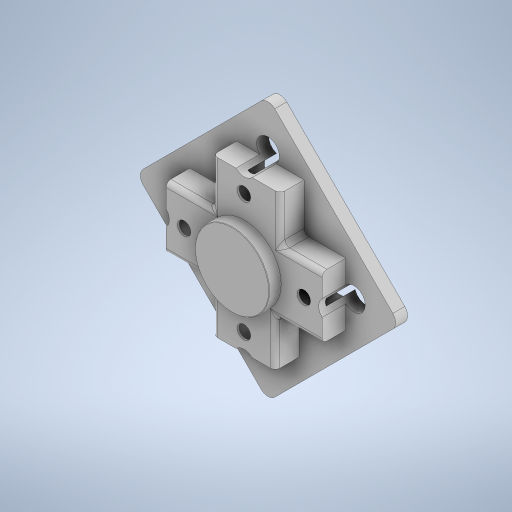
# Autodesk Inventor part: adapter_final2
Saved by Autodesk Inventor 2024 (Build 280153000, 153)
## iProperties
Created: 2024-05-24
Part Number: adapter_final2
Material: Generic
Document SubType Name: Modeling
Designer: maint
Density: 1 g/cm^3
Appearance: Default
Author: maint
Autodesk Inventor part; units mm, degrees
ref_plane "YZ Plane" through (0, 0, 0) normal (1, 0, 0) x (0, 1, 0)
ref_plane "XZ Plane" through (0, 0, 0) normal (0, 1, 0) x (-1, 0, 0)
ref_plane "XY Plane" through (0, 0, 0) normal (0, 0, 1) x (1, 0, 0)
sketch "Sketch1" plane through (0, 0, 0) normal (0, 0, 1) x (1, 0, 0)
  line L0 (41, -41) -> (-41, -41)
  line L1 (-41, -41) -> (-41, 41)
  line L2 (-41, 41) -> (41, 41)
  line L3 (41, 41) -> (41, -41)
  line L4 (41, -41) -> (-41, 41) construction
  line L5 (-41, -41) -> (41, 41) construction
  line L6 (-55, 0) -> (0, 55)
  line L7 (0, 55) -> (55, 0)
  line L8 (55, 0) -> (0, -55)
  line L9 (0, -55) -> (-55, 0)
  line L10 (-55, 0) -> (55, 0)
  line L11 (0, 55) -> (0, -55)
  circle A0 centre (0, 0) radius 63.5
  point P0 (-41, 0)
  dimension "d0" = 82
  dimension "d86" = 110
  dimension "d87" = 0
  dimension "d88" = 110
  dimension "d89" = 0
  dimension "d93" = 127
  constraints: 24 end point, 4 midpoint, 4 parallel, 3 perpendicular, 1 centre point, 1 coincident, 1 horizontal
  measures "d0" distance of L1.end L2.end
  measures "d86" distance of L8.end L6.end
  measures "d87" vertical distance of L7.end L6.start
  measures "d88" distance of L7.end L6.start
  measures "d89" distance from line of point (-41, 0) L10
  measures "d93" diameter of A0
extrude "Extrusion1" add sketch "Sketch1" along normal blind 15 contours L8 L11 L0 | L0 L11 L10 L3 L8 | L3 L10 L8 | L11 L9 L0 | L0 L9 L1 L10 L11 | L10 L11 L2 L7 L3 | L3 L7 L10 | L10 L1 L6 L2 L11 | L9 L10 L1 | L10 L6 L1 | L11 L7 L2 | L2 L6 L11
sketch "Sketch2" plane through (0, 0, 0) normal (0, 0, -1) x (-1, 0, 0)
  arc A0 (41, 38) -> (38, 41) centre (38, 38) ccw
  line L0 (25.4, -25.4) -> (-25.4, -25.4)
  line L1 (-25.4, -25.4) -> (-25.4, 25.4)
  line L2 (-25.4, 25.4) -> (25.4, 25.4)
  line L3 (25.4, 25.4) -> (25.4, -25.4)
  line L4 (25.4, -25.4) -> (-25.4, 25.4) construction
  line L5 (-25.4, -25.4) -> (25.4, 25.4) construction
  circle A1 centre (-25.4, 25.4) radius 3.3
  circle A2 centre (25.4, 25.4) radius 3.3
  circle A3 centre (25.4, -25.4) radius 3.3
  circle A4 centre (-25.4, -25.4) radius 3.3
  circle A5 centre (35.921, 0) radius 3.35
  circle A6 centre (-35.921, 0) radius 3.35
  circle A7 centre (-0.0342, 35.921) radius 3.35
  circle A8 centre (-0.0342, -35.921) radius 3.35
  point P0 (0, 0)
  point P1 (40.1213, 40.1213)
  dimension "d32" = 50.8
  dimension "d33" = 6.6
  dimension "d60" = 6.7
  dimension "d61" = 35.921
  dimension "d62" = 6.7
  dimension "d63" = 35.921
  dimension "d65" = 6.7
  dimension "d66" = 6.7
  dimension "d67" = 35.921
  dimension "d68" = 35.921
  constraints: 12 end point, 9 centre point, 4 coincident, 3 equal radius, 3 point on circle, 2 midpoint, 2 parallel, 2 perpendicular, 1 horizontal
  measures "d32" distance of L1.end L2.end
  measures "d33" diameter of A2
  measures "d60" diameter of A5
  measures "d61" distance of A5.centre point (0, 0)
  measures "d62" diameter of A6
  measures "d63" distance of point (0, 0) A6.centre
  measures "d65" diameter of A7
  measures "d66" diameter of A8
  measures "d67" distance of point (0, 0) A7.centre
  measures "d68" distance of point (0, 0) A8.centre
hole "Hole3" at (0.0342, 35.921, 0) at (0.0342, -35.921, 0) at (35.921, 0, 0) at (-35.921, 0, 0) direction (0, 0, 1) diameter 6.6 end through all
sketch "Sketch3" plane through (0, 0, 0) normal (0, 0, -1) x (-1, 0, 0)
  circle A0 centre (0, 0) radius 31.5
  circle A1 centre (0, 0) radius 25
  circle A2 centre (0, 25) radius 2.7
  circle A3 centre (25, 0) radius 2.7
  circle A4 centre (0, -25) radius 2.7
  circle A5 centre (-25, 0) radius 2.7
  dimension "d7" = 63
  dimension "d12" = 5.4
  constraints: 6 centre point, 4 point on circle, 3 equal radius, 2 coincident
  measures "d7" diameter of A0
  measures "d12" diameter of A2
hole "Hole1" at (25, 0, 0) at (0, 25, 0) at (0, -25, 0) at (-25, 0, 0) direction (0, 0, 1) diameter 5.6 end through all
sketch "Sketch5" plane through (0, 0, 15) normal (0, 0, 1) x (1, 0, 0)
  circle A0 centre (0, 0) radius 15.5
  dimension "d44" = 31
  constraints: 1 centre point, 1 coincident
  measures "d44" diameter of A0
extrude "Extrusion3" add sketch "Sketch5" along normal blind 5
fillet "Fillet2" radius 0.2 1 edges at (-15.5, 0, 20)
sketch "Sketch6" plane through (0, 0, 15) normal (0, 0, 1) x (1, 0, 0)
  line L0 (38, 41) -> (-38, 41) projected
  line L1 (43.0859, 13) -> (15.0859, 13)
  line L2 (15.0859, 13) -> (15.0859, 41)
  line L3 (15.0859, 41) -> (43.0859, 41)
  line L4 (43.0859, 41) -> (43.0859, 13)
  line L5 (-38, -41) -> (38, -41) projected
  line L6 (41, -38) -> (41, 38) projected
  line L7 (13, -41) -> (41, -41)
  line L8 (41, -41) -> (41, -13)
  line L9 (41, -13) -> (13, -13)
  line L10 (13, -13) -> (13, -41)
  line L11 (-41, 38) -> (-41, -38) projected
  line L12 (-41, 13) -> (-13, 13)
  line L13 (-13, 13) -> (-13, 41)
  line L14 (-13, 41) -> (-41, 41)
  line L15 (-41, 41) -> (-41, 13)
  line L16 (-41, -13) -> (-13, -13)
  line L17 (-13, -13) -> (-13, -41)
  line L18 (-13, -41) -> (-41, -41)
  line L19 (-41, -41) -> (-41, -13)
  line L20 (-32.6, 13) -> (-41, 13)
  line L21 (-41, 13) -> (-41, -13)
  line L22 (-41, -13) -> (-32.6, -13)
  line L23 (-32.6, -13) -> (-32.6, 13)
  line L24 (-13, -41) -> (13, -41)
  line L25 (13, -41) -> (13, -32.6)
  line L26 (13, -32.6) -> (-13, -32.6)
  line L27 (-13, -32.6) -> (-13, -41)
  line L28 (41, -13) -> (32.6, -13)
  line L29 (32.6, -13) -> (32.6, 13)
  line L30 (32.6, 13) -> (41, 13)
  line L31 (41, 13) -> (41, -13)
  line L32 (15.0859, 41) -> (-13, 41)
  line L33 (-13, 41) -> (-13, 32.6)
  line L34 (-13, 32.6) -> (15.0859, 32.6)
  line L35 (15.0859, 32.6) -> (15.0859, 41)
  point P0 (0, 0)
  point P1 (41, 38)
  point P2 (-41, -13)
  point P3 (15.0859, 32.6)
  point P4 (-32.6, -13)
  point P5 (41, 13)
  dimension "d48" = 28
  dimension "d69" = 8.4
  dimension "d70" = 8.4
  dimension "d71" = 8.4
  dimension "d72" = 8.4
  constraints: 62 end point, 15 parallel, 11 point on line, 8 horizontal, 8 perpendicular, 6 equal length, 1 vertical, 5 other
  measures "d48" distance of L1.start L1.end
  measures "d69" distance between parallel lines of L23 L11
  measures "d71" distance between parallel lines of L0 L34
  measures "d72" distance between parallel lines of L5 L26
extrude "Extrusion4" cut sketch "Sketch6" against normal blind 10 contours L3 L4 L1 L2 L0 | L2 L34 L13 L0 | L13 L12 L11 L15 L14 L0 | L6 L9 L29 L1 | L6 L8 L7 L5 L10 L9 | L23 L16 L11 L12 | L16 L17 L5 L18 L19 L11 | L10 L5 L17 L26
fillet "Fillet3" radius 2 9 edges at (22.8, -13, 15) (23.8429, 13, 15) (41.5, 13, 15) (15.0859, 22.8, 15) (-13, 22.8, 15) (-13, -22.8, 15) (13, -22.8, 15) (-22.8, -13, 15) (-22.8, 13, 15)
fillet "Fillet4" radius 2 8 edges at (15.0859, 13, 9) (14.5001, 12.4142, 14.4142) (-13, 13, 9) (-12.4142, 12.4142, 14.4142) (13, -13, 9) (12.4142, -12.4142, 14.4142) (-13, -13, 9) (-12.4142, -12.4142, 14.4142)
sketch "Sketch8" plane through (0, 0, 0) normal (0, 0, -1) x (-1, 0, 0)
  circle A0 centre (0, 0) radius 25.0495
  circle A1 centre (0, 25.0495) radius 6.4625
  circle A2 centre (25.0495, 0) radius 6.4505
  circle A3 centre (0, -25) radius 6.5 projected
  circle A4 centre (0, -25) radius 6.5
  circle A5 centre (-25.0495, 0) radius 6.5495
  constraints: 5 centre point, 3 point on circle, 2 coincident
hole "Hole4" at (0, -25, 0) at (-25.0495, 0, 0) at (0, 25.0495, 0) at (25.0495, 0, 0) direction (0, 0, 1) diameter 13 depth 12 tip angle 118
sketch "Sketch9" plane through (0, 0, 15) normal (0, 0, 1) x (1, 0, 0)
  circle A0 centre (0.0342, 35.921) radius 3.3 projected
  arc A1 (-0.0024, 31.2413) -> (0.0342, 31.2412) centre (0.0342, 35.921) ccw
  circle A2 centre (0.0342, 35.921) radius 4.75
  circle A3 centre (35.921, 0) radius 3.3 projected
  circle A4 centre (35.921, 0) radius 4.75
  circle A5 centre (0.0342, -35.921) radius 3.3 projected
  circle A6 centre (0.0342, -35.921) radius 4.75
  circle A7 centre (-35.921, 0) radius 3.3 projected
  circle A8 centre (-35.921, 0) radius 4.75
  point P0 (0, 0)
  dimension "d80" = 9.5
  dimension "d83" = 9.5
  dimension "d84" = 9.5
  dimension "d85" = 9.5
  constraints: 5 centre point, 5 coincident, 2 point on circle
  measures "d80" diameter of A2
  measures "d83" diameter of A4
  measures "d84" diameter of A6
  measures "d85" diameter of A8
hole "Hole5" at (0.0342, 35.921, 15) at (0.0342, -35.921, 15) at (35.921, 0, 15) at (-35.921, 0, 15) direction (0, 0, -1) diameter 9.5 depth 15
fillet "Fillet5" radius 4 4 edges at (0, 55, 7.5) (55, 0, 7.5) (-55, 0, 7.5) (0, -55, 7.5)
sketch "Sketch10" plane through (0, 0, 15) normal (0, 0, 1) x (1, 0, 0)
  line L0 (-41, -14) -> (-41, 14) projected
  line L1 (-41, 14) -> (-41, -14)
  line L2 (-41, -14) -> (-55, 0)
  line L3 (-52.1716, -2.8284) -> (-2.8284, -52.1716) projected
  line L4 (-55, 0) -> (-41, 14)
  line L5 (2.8284, -52.1716) -> (14, -41) projected
  line L6 (14, -41) -> (-14, -41)
  line L7 (41, -14) -> (52.1716, -2.8284) projected
  line L8 (41, -14) -> (55, 0)
  line L9 (14, 41) -> (42, 13) projected
  line L10 (55, 0) -> (41, 14)
  line L11 (41, -14) -> (41, 14)
  line L12 (-14, 41) -> (14, 41) projected
  line L13 (-14, 41) -> (14, 41)
  line L14 (14, 41) -> (0, 55)
  line L15 (0, 55) -> (-14, 41)
  line L16 (14, -41) -> (-14, -41)
  line L17 (0, -55) -> (-14, -41)
  line L18 (14, -41) -> (0, -55)
  point P0 (0, 0)
  point P1 (43.0859, 14.8971)
  point P2 (43.0859, 14.8971)
  point P3 (42, 13)
  constraints: 26 end point, 4 collinear, 2 perpendicular, 2 point on line, 1 horizontal, 1 vertical, 3 other
extrude "Extrusion5" cut sketch "Sketch10" against normal blind 10
equation "\"d63\" = d61"
equation "\"d67\" = d61"
equation "\"d68\" = d61"
equation "\"d70\" = d69"
equation "\"d71\" = d69"
equation "\"d72\" = d69"
equation "\"d83\" = d80"
equation "\"d84\" = d80"
equation "\"d85\" = d80"
equation "\"d73\" = d85"
body "Solid1"
